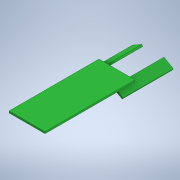
# Autodesk Inventor part: buttons_PCBs
Saved by Autodesk Inventor 2020 (Build 240168000, 168)
## iProperties
Created: 2019-11-16
Part Number: buttons_PCBs
Material: Generic
Document SubType Name: Modeling
Designer: suchanek
Density: 1 g/cm^3
Appearance: Default
Author: suchanek
Autodesk Inventor part; units mm, degrees
ref_plane "YZ Plane" through (0, 0, 0) normal (1, 0, 0) x (0, 1, 0)
ref_plane "XZ Plane" through (0, 0, 0) normal (0, 1, 0) x (-1, 0, 0)
ref_plane "XY Plane" through (0, 0, 0) normal (0, 0, 1) x (1, 0, 0)
sketch "Sketch1" plane through (0, 0, 0) normal (0, 0, 1) x (1, 0, 0)
  line L0 (0, 0) -> (20, 0)
  line L1 (20, 0) -> (20, 1)
  line L2 (20, 1) -> (0, 1)
  line L3 (0, 1) -> (0, 0)
  dimension "d0" = 20
  dimension "d1" = 1
  constraints: 8 end point, 2 parallel, 1 horizontal, 1 perpendicular
  measures "d0" distance of L2.end L1.end
  measures "d1" distance of L1.end L0.end
extrude "Extrusion1" add sketch "Sketch1" along normal blind 50
sketch "Sketch2" plane through (0, 0, 0) normal (0, 0, -1) x (-1, 0, 0)
  line L0 (0, 0) -> (-20, 0) projected
  line L1 (-3.8175, 0) -> (1.3787, -3)
  line L2 (1.3787, -3) -> (0.8787, -3.866)
  line L3 (0.8787, -3.866) -> (-4.3175, -0.866)
  line L4 (-4.3175, -0.866) -> (-3.8175, 0)
  line L5 (-10, 0) -> (-10, -4.6916)
  line L6 (-16.1825, 0) -> (-21.3787, -3)
  line L7 (-21.3787, -3) -> (-20.8787, -3.866)
  line L8 (-20.8787, -3.866) -> (-15.6825, -0.866)
  line L9 (-15.6825, -0.866) -> (-16.1825, 0)
  dimension "d4" = 1
  dimension "d6" = 12.365
  dimension "d7" = 120
  dimension "d8" = 6
  constraints: 18 end point, 4 symmetric about line, 2 parallel, 1 midpoint, 1 perpendicular, 1 point on line, 1 vertical
  measures "d4" distance of L1.end L2.end
  measures "d6" distance of L1.start L6.start
  measures "d7" angle of L3 L8
  measures "d8" distance of L1.start L1.end
extrude "Extrusion2" add sketch "Sketch2" along normal blind 20 and the other way blind 8
body "Solid1"
